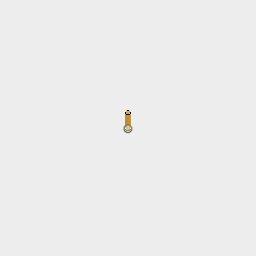
leg_Part_2 (Autodesk Fusion 360 design; units mm, degrees)
Autodesk Fusion 360 part; units mm, degrees
cylinder "CylinderPrimitive1" add diameter 10 height 35 placed x (1, 0, 0) y (0, 0, -1) z (0, 1, 0) at (0, 0, 0) makes body 1
sketch "sketch 1910" plane through (0, 0, 0) normal (0, 0, 1) x (1, 0, 0)
  line L0 (0, 0) -> (5, 0)
  arc A0 (5, 0) -> (1.4, 4.8) centre (0, 0) ccw
  line L1 (0, 4.8) -> (1.4, 4.8)
  line L2 (0, 0) -> (0, 4.8)
revolve "Revolve1" add sketch "sketch 1910" angle 360 about axis through (0, 205.75, 0) along (0, -1, 0) separate body makes body 2 in component "leg_1_Part_2_bottom"
sketch "sketch 1945" plane through (0, 0, 0) normal (0, 0, 1) x (1, 0, 0)
  line L0 (0, 0) -> (5, 0)
  arc A0 (5, 0) -> (1.4, 4.8) centre (0, 0) ccw
  line L1 (0, 4.8) -> (1.4, 4.8)
  line L2 (0, 0) -> (0, 4.8)
revolve "Revolve1'" add sketch "sketch 1945" angle 360 about axis through (0, -240.75, 0) along (0, 1, 0) separate body makes body 3 in component "leg_1_Part_2_top"
component "leg_1_Part_2_bottom" placed x (1, 0, 0) y (0, -1, 0) z (0, 0, -1) at (0, 0, 0)
component "leg_1_Part_2_top" placed x (1, 0, 0) y (0, 1, 0) z (0, 0, 1) at (0, 35, 0)
